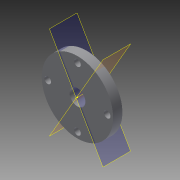
# Autodesk Inventor part: 零件7-18
Saved by Autodesk Inventor 2014 (Build 180170000, 170)
## iProperties
Created: 2018-12-21
Part Number: 零件7-18
Material: 常规
Document SubType Name: Modeling
Designer: Administrator
Density: 1 g/cm^3
Appearance: 默认
Author: Administrator
Autodesk Inventor part; units mm, degrees
ref_plane "YZ Plane" through (0, 0, 0) normal (1, 0, 0) x (0, 1, 0)
ref_plane "XZ Plane" through (0, 0, 0) normal (0, 1, 0) x (-1, 0, 0)
sketch "草图1" plane through (0, 0, 0) normal (0, 1, 0) x (-1, 0, 0)
  circle A0 centre (0, 0) radius 27
  circle A1 centre (0, 0) radius 22.5 construction
  circle A2 centre (22.5, 0) radius 2.5
  circle A3 centre (0, -22.5) radius 2.5
  circle A4 centre (-22.5, 0) radius 2.5
  circle A5 centre (0, 22.5) radius 2.5
  dimension "d0" = 54
  dimension "d1" = 45
  dimension "d2" = 5
  dimension "d3" = 5
  dimension "d4" = 5
  dimension "d5" = 5
  constraints: 6 centre point, 4 point on circle, 2 coincident
  measures "d0" diameter of A0
  measures "d1" diameter of A1
  measures "d2" diameter of A2
  measures "d3" diameter of A3
  measures "d4" diameter of A4
  measures "d5" diameter of A5
extrude "拉伸1" add sketch "草图1" along normal blind 7
sketch "草图2" plane through (0, 7, 0) normal (0, 1, 0) x (1, 0, 0)
  circle A0 centre (0, 0) radius 27 projected
  circle A1 centre (0, 0) radius 10
  dimension "d8" = 20
  constraints: 1 centre point, 1 coincident
  measures "d8" diameter of A1
extrude "拉伸2" add sketch "草图2" along normal blind 12 contours A1
sketch "草图3" plane through (0, 19, 0) normal (0, 1, 0) x (1, 0, 0)
  circle A0 centre (0, 0) radius 10 projected
  circle A1 centre (0, 0) radius 6
  dimension "d11" = 12
  constraints: 1 centre point, 1 coincident
  measures "d11" diameter of A1
extrude "拉伸3" cut sketch "草图3" against normal blind 19 contours A1
sketch "草图4" plane through (0, 0, 0) normal (0, 0, 1) x (1, 0, 0)
  line L0 (10, 19) -> (-10, 19) projected
  line L1 (-10, 7) -> (10, 7) projected
  line L2 (27, 7) -> (-27, 7) projected
  line L3 (-27, 0) -> (27, 0) projected
  line L4 (8.6752, 19) -> (8.6752, 7)
  line L5 (8.6752, 19) -> (18.2273, 7)
  line L6 (8.6752, 7) -> (18.2273, 7)
  point P0 (0, 0)
  constraints: 6 end point, 3 point on line, 2 perpendicular
extrude "拉伸4" add sketch "草图4" along normal mid plane 6
ref_plane "工作平面1" through (0, 19, 0) normal (-0.866, 0, -0.5) x (0, -1, 0)
sketch "草图5" plane through (0, 19, 0) normal (-0.866, 0, -0.5) x (0, -1, 0)
  point P0 (19, 0)
sketch "草图6" plane through (0, 19, 0) normal (-0.866, 0, -0.5) x (0, -1, 0)
  point P0 (19, 0)
sketch "草图7" plane through (0, 19, 0) normal (-0.866, 0, -0.5) x (0, -1, 0)
  line L0 (12, -2.1716) -> (1.0857, -2.1716) projected
  ellipse E0 centre (-10.8983, 0) end of major axis (-22.7486, 7.5911) minor radius 7.7307 (1.0857, -7.3678) -> (1.0857, -2.1716) ccw projected
  line L1 (1.0857, -7.3678) -> (12, -7.3678) projected
  line L2 (12, -2.1716) -> (12, -7.3678) projected
  line L3 (0, 10) -> (0, -10) projected
  line L4 (12, 27) -> (12, -27) projected
  line L5 (19, -27) -> (19, 27) projected
  line L6 (0, 8.0111) -> (12, 8.0111)
  line L7 (12, 18.564) -> (0, 8.0111)
  line L8 (12, 18.564) -> (12, 8.0111)
  point P0 (19, 0)
  constraints: 6 end point, 3 point on line, 1 collinear, 1 perpendicular, 1 other
extrude "拉伸5" add sketch "草图7" along normal mid plane 6 contours L6 L7 L4
ref_plane "工作平面2" through (0, 19, 0) normal (0.866, 0, -0.5) x (0, -1, 0)
sketch "草图8" plane through (0, 19, 0) normal (0.866, 0, -0.5) x (0, -1, 0)
  line L0 (0, 10) -> (0, -10) projected
  line L1 (12, -2.1716) -> (1.7379, -2.1716) projected
  ellipse E0 centre (-9.1096, 0) end of major axis (1.2979, -8.0654) minor radius 7.4792 (1.7379, -7.3678) -> (1.7379, -2.1716) ccw projected
  line L2 (1.7379, -7.3678) -> (12, -7.3678) projected
  line L3 (12, -7.3678) -> (12, -7.3678) projected
  line L4 (12, -7.3678) -> (1.0857, -7.3678) projected
  ellipse E1 centre (-10.8983, 0) end of major axis (-22.7486, 7.5911) minor radius 7.7307 (1.0857, -7.3678) -> (1.0857, -2.1716) ccw projected
  line L5 (1.0857, -2.1716) -> (12, -2.1716) projected
  line L6 (12, -2.1716) -> (12, -2.1716) projected
  line L7 (12, 27) -> (12, -27) projected
  line L8 (19, -27) -> (19, 27) projected
  line L9 (0, 6.3008) -> (12, 6.3008)
  line L10 (0, 6.3008) -> (12, 15.6151)
  line L11 (12, 15.6151) -> (12, 6.3008)
  point P0 (19, 0)
  constraints: 6 end point, 3 point on line, 1 collinear, 1 perpendicular, 2 other
extrude "拉伸6" add sketch "草图8" along normal mid plane 6 contours L9 L10 L7
